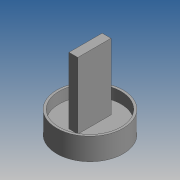
# Autodesk Inventor part: P011_Chapeau_chambre
Saved by Autodesk Inventor 2021.4 (Build 254397000, 397)
## iProperties
Created: 2022-03-24
Part Number: P011_Chapeau_chambre
Material: Générique
Document SubType Name: Modeling
Designer: Maintenant Prêt
Density: 1 g/cm^3
Appearance: Par défaut
Author: Maintenant Prêt
Autodesk Inventor part; units mm, degrees
ref_plane "YZ Plane" through (0, 0, 0) normal (1, 0, 0) x (0, 1, 0)
ref_plane "XZ Plane" through (0, 0, 0) normal (0, 1, 0) x (-1, 0, 0)
ref_plane "XY Plane" through (0, 0, 0) normal (0, 0, 1) x (1, 0, 0)
sketch "Sketch2" plane through (0, 0, 0) normal (0, 0, 1) x (1, 0, 0)
  line L0 (-21, 0) -> (21, 0) construction
  line L1 (0, -21) -> (0, 21) construction
  circle A0 centre (0, 0) radius 15
  dimension "d0" = 30
  constraints: 1 centre point, 1 coincident
  measures "d0" diameter of A0
extrude "Extrusion1" add sketch "Sketch2" along normal blind 5
sketch "Sketch3" plane through (0, 0, 5) normal (0, 0, 1) x (1, 0, 0)
  line L0 (-21, 0) -> (21, 0) construction
  line L1 (0, -21) -> (0, 21) construction
  line L2 (-2, 7.5) -> (2, 7.5)
  line L3 (2, 7.5) -> (2, -7.5)
  line L4 (2, -7.5) -> (-2, -7.5)
  line L5 (-2, -7.5) -> (-2, 7.5)
  point P0 (0, 0)
  dimension "d3" = 2
  dimension "d5" = 15
  constraints: 8 end point, 2 parallel, 1 horizontal, 1 perpendicular, 2 other
  measures "d3" distance between parallel lines of L3 L1
  measures "d5" distance between parallel lines of L4 L2
extrude "Extrusion2" add sketch "Sketch3" along normal blind 30
sketch "Sketch4" plane through (0, 0, 5) normal (0, 0, 1) x (1, 0, 0)
  circle A0 centre (0, 0) radius 15 construction
  line L0 (0, -21) -> (0, 21) construction
  line L1 (-21, 0) -> (21, 0) construction
  circle A1 centre (0, 0) radius 14
  circle A2 centre (0, 0) radius 15
  dimension "d8" = 28
  constraints: 2 centre point, 2 coincident, 1 concentric
  measures "d8" diameter of A1
extrude "Extrusion3" add sketch "Sketch4" along normal blind 5
body "Solid1"
